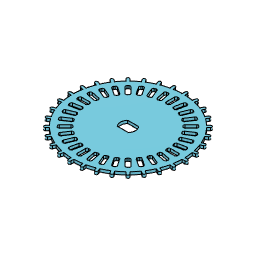
feeder-rev03 (Autodesk Fusion 360 archive; units mm, degrees)
design "indexingWheel"
Autodesk Fusion 360 part; units mm, degrees
sketch "Sketch1" plane through (0, 0, 0) normal (0, 1, 0) x (1, 0, 0)
  circle A0 centre (0, 0) radius 20
  circle A1 centre (0, 21) radius 0.5
  line L0 (2.5, 0) -> (20, 0)
  line L1 (0, -20) -> (0, -2.5)
  line L2 (-0.5, 21) -> (-0.5, 19.9937)
  line L3 (0.5, 21) -> (0.5, 19.9937)
  circle A2 centre (-4.0969, 20.5965) radius 0.5
  line L4 (-4.5873, 20.4989) -> (-4.391, 19.512)
  line L5 (-3.6065, 20.694) -> (-3.4102, 19.7071)
  circle A3 centre (-8.0364, 19.4015) radius 0.5
  line L6 (-8.4983, 19.2101) -> (-8.1132, 18.2805)
  line L7 (-7.5744, 19.5928) -> (-7.1893, 18.6632)
  circle A4 centre (-11.667, 17.4609) radius 0.5
  line L8 (-12.0827, 17.1831) -> (-11.5237, 16.3464)
  line L9 (-11.2512, 17.7386) -> (-10.6922, 16.902)
  circle A5 centre (-14.8492, 14.8492) radius 0.5
  line L10 (-15.2028, 14.4957) -> (-14.4913, 13.7842)
  line L11 (-14.4957, 15.2028) -> (-13.7842, 14.4913)
  circle A6 centre (-17.4609, 11.667) radius 0.5
  line L12 (-17.7386, 11.2512) -> (-16.902, 10.6922)
  line L13 (-17.1831, 12.0827) -> (-16.3464, 11.5237)
  circle A7 centre (-19.4015, 8.0364) radius 0.5
  line L14 (-19.5928, 7.5744) -> (-18.6632, 7.1893)
  line L15 (-19.2101, 8.4983) -> (-18.2805, 8.1132)
  circle A8 centre (-20.5965, 4.0969) radius 0.5
  line L16 (-20.694, 3.6065) -> (-19.7071, 3.4102)
  line L17 (-20.4989, 4.5873) -> (-19.512, 4.391)
  circle A9 centre (-21, 0) radius 0.5
  line L18 (-21, -0.5) -> (-19.9937, -0.5)
  line L19 (-21, 0.5) -> (-19.9937, 0.5)
  circle A10 centre (-20.5965, -4.0969) radius 0.5
  line L20 (-20.4989, -4.5873) -> (-19.512, -4.391)
  line L21 (-20.694, -3.6065) -> (-19.7071, -3.4102)
  circle A11 centre (-19.4015, -8.0364) radius 0.5
  line L22 (-19.2101, -8.4983) -> (-18.2805, -8.1132)
  line L23 (-19.5928, -7.5744) -> (-18.6632, -7.1893)
  circle A12 centre (-17.4609, -11.667) radius 0.5
  line L24 (-17.1831, -12.0827) -> (-16.3464, -11.5237)
  line L25 (-17.7386, -11.2512) -> (-16.902, -10.6922)
  circle A13 centre (-14.8492, -14.8492) radius 0.5
  line L26 (-14.4957, -15.2028) -> (-13.7842, -14.4913)
  line L27 (-15.2028, -14.4957) -> (-14.4913, -13.7842)
  circle A14 centre (-11.667, -17.4609) radius 0.5
  line L28 (-11.2512, -17.7386) -> (-10.6922, -16.902)
  line L29 (-12.0827, -17.1831) -> (-11.5237, -16.3464)
  circle A15 centre (-8.0364, -19.4015) radius 0.5
  line L30 (-7.5744, -19.5928) -> (-7.1893, -18.6632)
  line L31 (-8.4983, -19.2101) -> (-8.1132, -18.2805)
  circle A16 centre (-4.0969, -20.5965) radius 0.5
  line L32 (-3.6065, -20.694) -> (-3.4102, -19.7071)
  line L33 (-4.5873, -20.4989) -> (-4.391, -19.512)
  circle A17 centre (0, -21) radius 0.5
  line L34 (0.5, -21) -> (0.5, -19.9937)
  line L35 (-0.5, -21) -> (-0.5, -19.9937)
  circle A18 centre (4.0969, -20.5965) radius 0.5
  line L36 (4.5873, -20.4989) -> (4.391, -19.512)
  line L37 (3.6065, -20.694) -> (3.4102, -19.7071)
  circle A19 centre (8.0364, -19.4015) radius 0.5
  line L38 (8.4983, -19.2101) -> (8.1132, -18.2805)
  line L39 (7.5744, -19.5928) -> (7.1893, -18.6632)
  circle A20 centre (11.667, -17.4609) radius 0.5
  line L40 (12.0827, -17.1831) -> (11.5237, -16.3464)
  line L41 (11.2512, -17.7386) -> (10.6922, -16.902)
  circle A21 centre (14.8492, -14.8492) radius 0.5
  line L42 (15.2028, -14.4957) -> (14.4913, -13.7842)
  line L43 (14.4957, -15.2028) -> (13.7842, -14.4913)
  circle A22 centre (17.4609, -11.667) radius 0.5
  line L44 (17.7386, -11.2512) -> (16.902, -10.6922)
  line L45 (17.1831, -12.0827) -> (16.3464, -11.5237)
  circle A23 centre (19.4015, -8.0364) radius 0.5
  line L46 (19.5928, -7.5744) -> (18.6632, -7.1893)
  line L47 (19.2101, -8.4983) -> (18.2805, -8.1132)
  circle A24 centre (20.5965, -4.0969) radius 0.5
  line L48 (20.694, -3.6065) -> (19.7071, -3.4102)
  line L49 (20.4989, -4.5873) -> (19.512, -4.391)
  circle A25 centre (21, 0) radius 0.5
  line L50 (21, 0.5) -> (19.9937, 0.5)
  line L51 (21, -0.5) -> (19.9937, -0.5)
  circle A26 centre (20.5965, 4.0969) radius 0.5
  line L52 (20.4989, 4.5873) -> (19.512, 4.391)
  line L53 (20.694, 3.6065) -> (19.7071, 3.4102)
  circle A27 centre (19.4015, 8.0364) radius 0.5
  line L54 (19.2101, 8.4983) -> (18.2805, 8.1132)
  line L55 (19.5928, 7.5744) -> (18.6632, 7.1893)
  circle A28 centre (17.4609, 11.667) radius 0.5
  line L56 (17.1831, 12.0827) -> (16.3464, 11.5237)
  line L57 (17.7386, 11.2512) -> (16.902, 10.6922)
  circle A29 centre (14.8492, 14.8492) radius 0.5
  line L58 (14.4957, 15.2028) -> (13.7842, 14.4913)
  line L59 (15.2028, 14.4957) -> (14.4913, 13.7842)
  circle A30 centre (11.667, 17.4609) radius 0.5
  line L60 (11.2512, 17.7386) -> (10.6922, 16.902)
  line L61 (12.0827, 17.1831) -> (11.5237, 16.3464)
  line L62 (-0.75, 14) -> (0.75, 14)
  line L63 (0.75, 14) -> (0.75, 18)
  line L64 (0.75, 18) -> (-0.75, 18)
  line L65 (-0.75, 18) -> (-0.75, 14)
  line L66 (-2.776, 17.8005) -> (-4.2472, 17.5078)
  line L67 (-4.2472, 17.5078) -> (-3.4669, 13.5847)
  line L68 (-3.4669, 13.5847) -> (-1.9957, 13.8773)
  line L69 (-1.9957, 13.8773) -> (-2.776, 17.8005)
  line L70 (-6.1954, 16.9168) -> (-7.5812, 16.3428)
  line L71 (-7.5812, 16.3428) -> (-6.0505, 12.6473)
  line L72 (-6.0505, 12.6473) -> (-4.6647, 13.2213)
  line L73 (-4.6647, 13.2213) -> (-6.1954, 16.9168)
  line L74 (-9.3767, 15.3831) -> (-10.6239, 14.5498)
  line L75 (-10.6239, 14.5498) -> (-8.4016, 11.2239)
  line L76 (-8.4016, 11.2239) -> (-7.1544, 12.0573)
  line L77 (-7.1544, 12.0573) -> (-9.3767, 15.3831)
  line L78 (-12.1976, 13.2583) -> (-13.2583, 12.1976)
  line L79 (-13.2583, 12.1976) -> (-10.4298, 9.3692)
  line L80 (-10.4298, 9.3692) -> (-9.3692, 10.4298)
  line L81 (-9.3692, 10.4298) -> (-12.1976, 13.2583)
  line L82 (-14.5498, 10.6239) -> (-15.3831, 9.3767)
  line L83 (-15.3831, 9.3767) -> (-12.0573, 7.1544)
  line L84 (-12.0573, 7.1544) -> (-11.2239, 8.4016)
  line L85 (-11.2239, 8.4016) -> (-14.5498, 10.6239)
  line L86 (-16.3428, 7.5812) -> (-16.9168, 6.1954)
  line L87 (-16.9168, 6.1954) -> (-13.2213, 4.6647)
  line L88 (-13.2213, 4.6647) -> (-12.6473, 6.0505)
  line L89 (-12.6473, 6.0505) -> (-16.3428, 7.5812)
  line L90 (-17.5078, 4.2472) -> (-17.8005, 2.776)
  line L91 (-17.8005, 2.776) -> (-13.8773, 1.9957)
  line L92 (-13.8773, 1.9957) -> (-13.5847, 3.4669)
  line L93 (-13.5847, 3.4669) -> (-17.5078, 4.2472)
  line L94 (-18, 0.75) -> (-18, -0.75)
  line L95 (-18, -0.75) -> (-14, -0.75)
  line L96 (-14, -0.75) -> (-14, 0.75)
  line L97 (-14, 0.75) -> (-18, 0.75)
  line L98 (-17.8005, -2.776) -> (-17.5078, -4.2472)
  line L99 (-17.5078, -4.2472) -> (-13.5847, -3.4669)
  line L100 (-13.5847, -3.4669) -> (-13.8773, -1.9957)
  line L101 (-13.8773, -1.9957) -> (-17.8005, -2.776)
  line L102 (-16.9168, -6.1954) -> (-16.3428, -7.5812)
  line L103 (-16.3428, -7.5812) -> (-12.6473, -6.0505)
  line L104 (-12.6473, -6.0505) -> (-13.2213, -4.6647)
  line L105 (-13.2213, -4.6647) -> (-16.9168, -6.1954)
  line L106 (-15.3831, -9.3767) -> (-14.5498, -10.6239)
  line L107 (-14.5498, -10.6239) -> (-11.2239, -8.4016)
  line L108 (-11.2239, -8.4016) -> (-12.0573, -7.1544)
  line L109 (-12.0573, -7.1544) -> (-15.3831, -9.3767)
  line L110 (-13.2583, -12.1976) -> (-12.1976, -13.2583)
  line L111 (-12.1976, -13.2583) -> (-9.3692, -10.4298)
  line L112 (-9.3692, -10.4298) -> (-10.4298, -9.3692)
  line L113 (-10.4298, -9.3692) -> (-13.2583, -12.1976)
  line L114 (-10.6239, -14.5498) -> (-9.3767, -15.3831)
  line L115 (-9.3767, -15.3831) -> (-7.1544, -12.0573)
  line L116 (-7.1544, -12.0573) -> (-8.4016, -11.2239)
  line L117 (-8.4016, -11.2239) -> (-10.6239, -14.5498)
  line L118 (-7.5812, -16.3428) -> (-6.1954, -16.9168)
  line L119 (-6.1954, -16.9168) -> (-4.6647, -13.2213)
  line L120 (-4.6647, -13.2213) -> (-6.0505, -12.6473)
  line L121 (-6.0505, -12.6473) -> (-7.5812, -16.3428)
  line L122 (-4.2472, -17.5078) -> (-2.776, -17.8005)
  line L123 (-2.776, -17.8005) -> (-1.9957, -13.8773)
  line L124 (-1.9957, -13.8773) -> (-3.4669, -13.5847)
  line L125 (-3.4669, -13.5847) -> (-4.2472, -17.5078)
  line L126 (-0.75, -18) -> (0.75, -18)
  line L127 (0.75, -18) -> (0.75, -14)
  line L128 (0.75, -14) -> (-0.75, -14)
  line L129 (-0.75, -14) -> (-0.75, -18)
  line L130 (2.776, -17.8005) -> (4.2472, -17.5078)
  line L131 (4.2472, -17.5078) -> (3.4669, -13.5847)
  line L132 (3.4669, -13.5847) -> (1.9957, -13.8773)
  line L133 (1.9957, -13.8773) -> (2.776, -17.8005)
  line L134 (6.1954, -16.9168) -> (7.5812, -16.3428)
  line L135 (7.5812, -16.3428) -> (6.0505, -12.6473)
  line L136 (6.0505, -12.6473) -> (4.6647, -13.2213)
  line L137 (4.6647, -13.2213) -> (6.1954, -16.9168)
  line L138 (9.3767, -15.3831) -> (10.6239, -14.5498)
  line L139 (10.6239, -14.5498) -> (8.4016, -11.2239)
  line L140 (8.4016, -11.2239) -> (7.1544, -12.0573)
  line L141 (7.1544, -12.0573) -> (9.3767, -15.3831)
  line L142 (12.1976, -13.2583) -> (13.2583, -12.1976)
  line L143 (13.2583, -12.1976) -> (10.4298, -9.3692)
  line L144 (10.4298, -9.3692) -> (9.3692, -10.4298)
  line L145 (9.3692, -10.4298) -> (12.1976, -13.2583)
  line L146 (14.5498, -10.6239) -> (15.3831, -9.3767)
  line L147 (15.3831, -9.3767) -> (12.0573, -7.1544)
  line L148 (12.0573, -7.1544) -> (11.2239, -8.4016)
  line L149 (11.2239, -8.4016) -> (14.5498, -10.6239)
  line L150 (16.3428, -7.5812) -> (16.9168, -6.1954)
  line L151 (16.9168, -6.1954) -> (13.2213, -4.6647)
  line L152 (13.2213, -4.6647) -> (12.6473, -6.0505)
  line L153 (12.6473, -6.0505) -> (16.3428, -7.5812)
  line L154 (17.5078, -4.2472) -> (17.8005, -2.776)
  line L155 (17.8005, -2.776) -> (13.8773, -1.9957)
  line L156 (13.8773, -1.9957) -> (13.5847, -3.4669)
  line L157 (13.5847, -3.4669) -> (17.5078, -4.2472)
  line L158 (18, -0.75) -> (18, 0.75)
  line L159 (18, 0.75) -> (14, 0.75)
  line L160 (14, 0.75) -> (14, -0.75)
  line L161 (14, -0.75) -> (18, -0.75)
  line L162 (17.8005, 2.776) -> (17.5078, 4.2472)
  line L163 (17.5078, 4.2472) -> (13.5847, 3.4669)
  line L164 (13.5847, 3.4669) -> (13.8773, 1.9957)
  line L165 (13.8773, 1.9957) -> (17.8005, 2.776)
  line L166 (16.9168, 6.1954) -> (16.3428, 7.5812)
  line L167 (16.3428, 7.5812) -> (12.6473, 6.0505)
  line L168 (12.6473, 6.0505) -> (13.2213, 4.6647)
  line L169 (13.2213, 4.6647) -> (16.9168, 6.1954)
  line L170 (15.3831, 9.3767) -> (14.5498, 10.6239)
  line L171 (14.5498, 10.6239) -> (11.2239, 8.4016)
  line L172 (11.2239, 8.4016) -> (12.0573, 7.1544)
  line L173 (12.0573, 7.1544) -> (15.3831, 9.3767)
  line L174 (13.2583, 12.1976) -> (12.1976, 13.2583)
  line L175 (12.1976, 13.2583) -> (9.3692, 10.4298)
  line L176 (9.3692, 10.4298) -> (10.4298, 9.3692)
  line L177 (10.4298, 9.3692) -> (13.2583, 12.1976)
  line L178 (10.6239, 14.5498) -> (9.3767, 15.3831)
  line L179 (9.3767, 15.3831) -> (7.1544, 12.0573)
  line L180 (7.1544, 12.0573) -> (8.4016, 11.2239)
  line L181 (8.4016, 11.2239) -> (10.6239, 14.5498)
  circle A31 centre (0, 0) radius 2.7
  line L182 (7.5812, 16.3428) -> (6.1954, 16.9168)
  line L183 (6.1954, 16.9168) -> (4.6647, 13.2213)
  line L184 (4.6647, 13.2213) -> (6.0505, 12.6473)
  line L185 (6.0505, 12.6473) -> (7.5812, 16.3428)
  line L186 (4.2472, 17.5078) -> (2.776, 17.8005)
  line L187 (2.776, 17.8005) -> (1.9957, 13.8773)
  line L188 (1.9957, 13.8773) -> (3.4669, 13.5847)
  line L189 (3.4669, 13.5847) -> (4.2472, 17.5078)
  circle A32 centre (8.0364, 19.4015) radius 0.5
  line L190 (7.5744, 19.5928) -> (7.1893, 18.6632)
  line L191 (8.4983, 19.2101) -> (8.1132, 18.2805)
  circle A33 centre (4.0969, 20.5965) radius 0.5
  line L192 (3.6065, 20.694) -> (3.4102, 19.7071)
  line L193 (4.5873, 20.4989) -> (4.391, 19.512)
  line L194 (-1.9666, 1.85) -> (1.9666, 1.85)
  line L195 (1.9666, 1.85) -> (1.9666, -1.85)
  line L196 (1.9666, -1.85) -> (-1.9666, -1.85)
  line L197 (-1.9666, -1.85) -> (-1.9666, 1.85)
  point P0 (0, 14)
  dimension "d1" = 1
  dimension "d2" = 40
  dimension "d3" = 21
  dimension "d5" = 360
  dimension "d6" = 1.5
  dimension "d7" = 4
  dimension "d8" = 14
  dimension "d10" = 360
  dimension "d13" = 5.4
  dimension "d233" = 3.7
  constraint coincident A0.centre A31.centre
  constraint coincident A1.centre L1
  constraint coincident A1 L2.start
  constraint coincident A0 L2.end
  constraint vertical L2
  constraint coincident A1 L3.start
  constraint coincident A0 L3.end
  constraint parallel L2 L3
  constraint tangent A1 L2
  constraint tangent A1 L3
  constraint horizontal L62
  constraint vertical L63
  constraint horizontal L64
  constraint vertical L65
  constraint midpoint L62 P0
  constraint coincident L1 P0
  constraint horizontal L194
  constraint vertical L195
  constraint horizontal L196
  constraint vertical L197
  constraint coincident A31 L195.end
  constraint coincident A31 L194.start
  constraint coincident A31 L194.end
  measures "d1" diameter of A1
  measures "d2" diameter of A0
  measures "d3" distance of A0.centre A1.centre
  measures "d6" distance of L63 L65
  measures "d7" distance of L62 L64
  measures "d8" distance of A0.centre L62
  measures "d13" diameter of A31
  measures "d233" distance of L194 L196
extrude "Extrude1" add sketch "Sketch1" along normal blind 1 contours A0 L0 L1 L126 L128 L129 L158 L159 L160 A31 | A0 A25 L50 L51 | A0 L0 L1 L126 L127 L128 L158 L160 L161 A31 | A0 A26 L52 L53 | A25 | A0 A24 L48 L49 | A26 | A24 | A0 A27 L54 L55 | A0 A23 L46 L47 | A31 L194 | A31 L196 | A27 | A23 | A0 A28 L56 L57 | A0 A22 L44 L45 | A28 | A22 | A0 A29 L58 L59 | A0 A21 L42 L43 | A0 A17 L34 L35 | A29 | A21 | A0 A30 L60 L61 | A0 A20 L40 L41 | A0 A16 L32 L33 | A17 | A0 A18 L36 L37 | A30 | A20 | A16 | A18 | A0 A32 L190 L191 | A0 A19 L38 L39 | A0 A15 L30 L31 | A32 | A19 | A15 | A0 A33 L192 L193 | A0 A14 L28 L29 | A33 | A14 | A0 A1 L2 L3 | A0 A13 L26 L27 | A1 | A13 | A0 A2 L4 L5 | A0 A12 L24 L25 | A2 | A12 | A0 A3 L6 L7 | A0 A11 L22 L23 | A3 | A11 | A0 A4 L8 L9 | A0 A10 L20 L21 | A4 | A10 | A0 A5 L10 L11 | A0 A9 L18 L19 | A5 | A9 | A0 A6 L12 L13 | A0 A8 L16 L17 | A6 | A8 | A0 A7 L14 L15 | A7 in component "tapeGear"
fillet "Fillet2" radius 0.5 4 edges at (-0.75, 0.5, -18) (0.75, 0.5, -18) (0.75, 0.5, -14) (-0.75, 0.5, -14) in component "tapeGear"
pattern_circular "C-Pattern2" count 32 over 360 about axis through (0, 0, 0) along (0, 1, 0) of 4 faces at (-0.54, 0.3333, -17.9073) (0.6119, 0.3333, -17.845) (-0.7494, 0.3333, -14.4762) (0.7494, 0.3333, -14.4762) in component "tapeGear"
component "tapeGear" placed x (1, 0, 0) y (0, 1, 0) z (0, 0, 1) at (0, 0, 0)

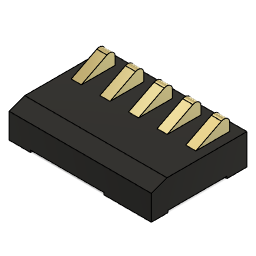
design "springFingers"
Autodesk Fusion 360 part; units mm, degrees
sketch "Sketch1" plane through (0, 0, 0) normal (0, 1, 0) x (1, 0, 0)
  line L0 (0, 0) -> (12.62, 0)
  line L1 (12.62, 0) -> (12.62, 8.48)
  line L2 (12.62, 8.48) -> (0, 8.48)
  line L3 (0, 8.48) -> (0, 0)
  dimension "d1" = 12.62
  dimension "d2" = 8.48
  constraint horizontal L0
  constraint vertical L1
  constraint horizontal L2
  constraint vertical L3
  constraint coincident L0.start L3.end
  measures "d1" distance of L0.start L0.end
  measures "d2" distance of L0.start L2.end
extrude "Extrude1" add sketch "Sketch1" along normal blind 2.54
chamfer "Chamfer1" distance 1.39 angle 20 1 edges at (6.31, 2.54, 0) measured on face at (4.2067, 2.54, -5.6533)
sketch "Sketch2" plane through (0, 2.54, 0) normal (0, 1, 0) x (-1, 0, 0)
  line L0 (0, -1.39) -> (-12.62, -1.39)
  line L1 (-12.62, -1.39) -> (-12.62, -8.48)
  line L2 (-12.62, -8.48) -> (0, -8.48)
  line L3 (0, -8.48) -> (0, -1.39)
  line L4 (-0.78, -7.73) -> (-1.68, -7.73)
  line L5 (-1.68, -7.73) -> (-1.68, -4.73)
  line L6 (-1.68, -4.73) -> (-0.78, -4.73)
  line L7 (-0.78, -4.73) -> (-0.78, -7.73)
  line L8 (-3.32, -4.73) -> (-3.32, -7.73)
  line L9 (-3.32, -7.73) -> (-4.22, -7.73)
  line L10 (-4.22, -7.73) -> (-4.22, -4.73)
  line L11 (-4.22, -4.73) -> (-3.32, -4.73)
  line L12 (-5.86, -4.73) -> (-5.86, -7.73)
  line L13 (-5.86, -7.73) -> (-6.76, -7.73)
  line L14 (-6.76, -7.73) -> (-6.76, -4.73)
  line L15 (-6.76, -4.73) -> (-5.86, -4.73)
  line L16 (-8.4, -4.73) -> (-8.4, -7.73)
  line L17 (-8.4, -7.73) -> (-9.3, -7.73)
  line L18 (-9.3, -7.73) -> (-9.3, -4.73)
  line L19 (-9.3, -4.73) -> (-8.4, -4.73)
  line L20 (-6.31, -8.48) -> (-6.31, -1.39) construction
  line L21 (-10.94, -4.73) -> (-10.94, -7.73)
  line L22 (-10.94, -7.73) -> (-11.84, -7.73)
  line L23 (-11.84, -7.73) -> (-11.84, -4.73)
  line L24 (-11.84, -4.73) -> (-10.94, -4.73)
  line L25 (-0.78, -7.73) -> (0, -7.73) construction
  line L26 (-11.84, -7.73) -> (-12.62, -7.73) construction
  dimension "d7" = 0.9
  dimension "d8" = 3
  dimension "d11" = -2.54
  dimension "d12" = 0
  dimension "d13" = 0.75
  constraint horizontal L4
  constraint vertical L5
  constraint horizontal L6
  constraint vertical L7
  constraint midpoint L2 L20.start
  constraint midpoint L0 L20.end
  constraint coincident L3 L25.end
  constraint perpendicular L3 L25
  constraint coincident L1 L26.end
  constraint perpendicular L1 L26
  constraint equal L25 L26
  measures "d7" distance of L4.start L4.end
  measures "d8" distance of L4.start L6.end
  measures "d13" distance of L2 L4
extrude "Extrude2" add sketch "Sketch2" along normal blind 1.27 contours L4 L5 L6 L7 | L8 L9 L10 L11 | L12 L13 L14 L15 | L16 L17 L18 L19 | L21 L22 L23 L24
chamfer "Chamfer2" distance 2.5 distance2 1.27 5 edges at (1.23, 3.81, -4.73) (3.77, 3.81, -4.73) (6.31, 3.81, -4.73) (8.85, 3.81, -4.73) (11.39, 3.81, -4.73) measured on face at (1.38, 3.81, -5.73) measured on face at (3.92, 3.81, -6.73) measured on face at (6.46, 3.81, -6.73) measured on face at (9, 3.81, -5.73) measured on face at (11.54, 3.81, -5.73)
fillet "Fillet1" radius 0.5 10 edges at (1.23, 3.81, -7.23) (1.23, 3.81, -7.73) (3.77, 3.81, -7.23) (3.77, 3.81, -7.73) (6.31, 3.81, -7.23) (6.31, 3.81, -7.73) (8.85, 3.81, -7.23) (8.85, 3.81, -7.73) (11.39, 3.81, -7.73) (11.39, 3.81, -7.23)
sketch "Sketch3" plane through (0, 0, 0) normal (0, -1, 0) x (1, 0, 0)
  line L0 (0, 0) -> (0, -8.48)
  line L1 (0, -8.48) -> (12.62, -8.48)
  line L2 (12.62, -8.48) -> (12.62, 0)
  line L3 (12.62, 0) -> (0, 0)
  line L4 (0, 0) -> (1.9102, 0)
  line L5 (1.9102, 0) -> (1.9102, -1.4751)
  line L6 (1.9102, -1.4751) -> (0, -1.4751)
  line L7 (0, -1.4751) -> (0, 0)
  line L8 (12.62, 0) -> (8.415, 0)
  line L9 (8.415, 0) -> (8.415, -1.4751)
  line L10 (8.415, -1.4751) -> (12.62, -1.4751)
  line L11 (12.62, -1.4751) -> (12.62, 0)
  line L12 (0, -8.48) -> (1.9102, -8.48)
  line L13 (1.9102, -8.48) -> (1.9102, -7.0162)
  line L14 (1.9102, -7.0162) -> (0, -7.0162)
  line L15 (0, -7.0162) -> (0, -8.48)
  line L16 (12.62, -8.48) -> (7.909, -8.48)
  line L17 (7.909, -8.48) -> (7.909, -6.703)
  line L18 (7.909, -6.703) -> (12.62, -6.703)
  line L19 (12.62, -6.703) -> (12.62, -8.48)
  constraint horizontal L4
  constraint vertical L5
  constraint horizontal L6
  constraint vertical L7
  constraint coincident L0.start L3.end
  constraint horizontal L8
  constraint vertical L9
  constraint horizontal L10
  constraint vertical L11
  constraint coincident L2.end L3.start
  constraint horizontal L12
  constraint vertical L13
  constraint horizontal L14
  constraint vertical L15
  constraint coincident L0.end L1.start
  constraint horizontal L16
  constraint vertical L17
  constraint horizontal L18
  constraint vertical L19
  constraint coincident L1.end L2.start
extrude "Extrude3" add sketch "Sketch3" along normal blind 0.18 contours L0 L3 L4 L5 L6 L7 | L0 L1 L12 L13 L14 L15 | L2 L3 L8 L9 L10 L11 | L1 L2 L16 L17 L18 L19
